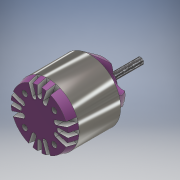
# Autodesk Inventor part: silnik
Saved by Autodesk Inventor 2017 (Build 210142000, 142)
## iProperties
Created: 2016-12-26
Part Number: silnik
Material: Ogólny
Document SubType Name: Modeling
Designer: Kuba01
Density: 1 g/cm^3
Appearance: Domyślna
Author: Kuba01
Autodesk Inventor part; units mm, degrees
ref_plane "YZ Plane" through (0, 0, 0) normal (1, 0, 0) x (0, 1, 0)
ref_plane "XZ Plane" through (0, 0, 0) normal (0, 1, 0) x (-1, 0, 0)
ref_plane "XY Plane" through (0, 0, 0) normal (0, 0, 1) x (1, 0, 0)
sketch "Szkic1" plane through (0, 0, 0) normal (0, 0, 1) x (1, 0, 0)
  line L0 (0, -24.0594) -> (0, 52.0933) projected
  line L1 (0, 38.3467) -> (0, -13.1804)
  line L2 (0, -4.7857) -> (-13, -4.7857)
  line L3 (-13, -4.7857) -> (-14, -0.7857)
  line L4 (-14, -0.7857) -> (-14, 18.2143)
  line L5 (-14, 18.2143) -> (-10, 24.2143)
  line L6 (-10, 24.2143) -> (-4.5, 24.2143)
  line L7 (-4.5, 26.2143) -> (-1.5, 26.2143)
  line L8 (-1.5, 26.2143) -> (-1.5, 41.2143)
  line L9 (-1.5, 41.2143) -> (0, 41.2143)
  line L10 (-4.5, 24.2143) -> (-4.5, 26.2143)
  point P0 (0, 0)
  dimension "d2" = 14
  dimension "d3" = 13
  dimension "d4" = 4
  dimension "d5" = 6
  dimension "d6" = 19
  dimension "d7" = 20
  dimension "d9" = 3
  dimension "d10" = 15
  dimension "d12" = 2
  dimension "d13" = 9
  constraints: 20 end point, 4 point on line, 3 perpendicular, 2 parallel, 1 horizontal, 1 vertical
  measures "d2" distance between parallel lines of L4 L0
  measures "d3" distance of L2.start L2.end
  measures "d4" distance from line of L3.end L2
  measures "d5" distance from line of L6 L4.end
  measures "d6" distance of L3.end L4.end
  measures "d7" diameter of L5.end L1
  measures "d9" diameter of L8 L1
  measures "d10" distance between parallel lines of L9 L7
  measures "d12" distance between parallel lines of L6 L7
  measures "d13" diameter of L10 L1
revolve "Obrót1" add sketch "Szkic1" angle 360 about axis through (0, 38.3467, 0) along (0, -1, 0)
sketch "Szkic2" plane through (0, -4.7857, 0) normal (0, -1, 0) x (1, 0, 0)
  arc A0 (-9, -1) -> (-9, 1) centre (-9, 0) ccw
  line L0 (-9, 1) -> (-12.9615, 1)
  line L1 (-9, -1) -> (-12.9615, -1)
  line L2 (0, 0) -> (-12.3693, 4) construction
  arc A1 (-7.9292, 1.5132) -> (-7.2946, 3.4099) centre (-7.6119, 2.4615) ccw
  line L3 (-12.6285, 3.0855) -> (-7.9292, 1.5132)
  line L4 (-7.2946, 3.4099) -> (-12.0058, 4.9861)
  line L5 (-22.3692, 0) -> (20.0615, 0) projected
  arc A2 (-7.2946, -3.4099) -> (-7.9292, -1.5132) centre (-7.6119, -2.4615) ccw
  line L6 (-12.6285, -3.0855) -> (-7.9292, -1.5132)
  line L7 (-7.2946, -3.4099) -> (-12.0058, -4.9861)
  line L8 (-3.4099, -7.2946) -> (-4.9861, -12.0058)
  arc A3 (-1.5132, -7.9292) -> (-3.4099, -7.2946) centre (-2.4615, -7.6119) ccw
  line L9 (-3.0855, -12.6285) -> (-1.5132, -7.9292)
  line L10 (-1, -9) -> (-1, -12.9615)
  arc A4 (1, -9) -> (-1, -9) centre (0, -9) ccw
  line L11 (1, -9) -> (1, -12.9615)
  line L12 (3.0855, -12.6285) -> (1.5132, -7.9292)
  arc A5 (3.4099, -7.2946) -> (1.5132, -7.9292) centre (2.4615, -7.6119) ccw
  line L13 (3.4099, -7.2946) -> (4.9861, -12.0058)
  line L14 (7.2946, -3.4099) -> (12.0058, -4.9861)
  arc A6 (7.9292, -1.5132) -> (7.2946, -3.4099) centre (7.6119, -2.4615) ccw
  line L15 (12.6285, -3.0855) -> (7.9292, -1.5132)
  line L16 (9, -1) -> (12.9615, -1)
  arc A7 (9, 1) -> (9, -1) centre (9, 0) ccw
  line L17 (9, 1) -> (12.9615, 1)
  line L18 (12.6285, 3.0855) -> (7.9292, 1.5132)
  arc A8 (7.2946, 3.4099) -> (7.9292, 1.5132) centre (7.6119, 2.4615) ccw
  line L19 (7.2946, 3.4099) -> (12.0058, 4.9861)
  line L20 (3.4099, 7.2946) -> (4.9861, 12.0058)
  arc A9 (1.5132, 7.9292) -> (3.4099, 7.2946) centre (2.4615, 7.6119) ccw
  line L21 (3.0855, 12.6285) -> (1.5132, 7.9292)
  line L22 (1, 9) -> (1, 12.9615)
  arc A10 (-1, 9) -> (1, 9) centre (0, 9) ccw
  line L23 (-1, 9) -> (-1, 12.9615)
  line L24 (-3.0855, 12.6285) -> (-1.5132, 7.9292)
  arc A11 (-3.4099, 7.2946) -> (-1.5132, 7.9292) centre (-2.4615, 7.6119) ccw
  line L25 (-3.4099, 7.2946) -> (-4.9861, 12.0058)
  arc A12 (-12.6285, -3.0855) -> (-12.5891, -3.2428) centre (0, 0) ccw
  arc A13 (-4.9861, -12.0058) -> (-3.0855, -12.6285) centre (0, 0) ccw
  arc A14 (-1, -12.9615) -> (1, -12.9615) centre (0, 0) ccw
  arc A15 (3.0855, -12.6285) -> (4.9861, -12.0058) centre (0, 0) ccw
  arc A16 (12.0058, -4.9861) -> (12.6285, -3.0855) centre (0, 0) ccw
  arc A17 (12.9615, -1) -> (12.9615, 1) centre (0, 0) ccw
  arc A18 (12.6285, 3.0855) -> (12.0058, 4.9861) centre (0, 0) ccw
  arc A19 (4.9861, 12.0058) -> (3.0855, 12.6285) centre (0, 0) ccw
  arc A20 (1, 12.9615) -> (-1, 12.9615) centre (0, 0) ccw
  arc A21 (-3.0855, 12.6285) -> (-4.9861, 12.0058) centre (0, 0) ccw
  line L26 (-12.0058, 4.9861) -> (-15.0727, 6.0122)
  line L27 (-15.0727, 6.0122) -> (-15.7072, 4.1156)
  line L28 (-15.7072, 4.1156) -> (-12.6285, 3.0855)
  line L29 (-12.9615, 1) -> (-16.3077, 1)
  line L30 (-16.3077, 1) -> (-16.3077, -1)
  line L31 (-16.3077, -1) -> (-12.9615, -1)
  line L32 (-12.6285, -3.0855) -> (-16.0368, -4.2258)
  line L33 (-16.0368, -4.2258) -> (-15.4022, -6.1225)
  line L34 (-15.4022, -6.1225) -> (-12.0058, -4.9861)
  dimension "d15" = 2
  dimension "d16" = 9
  dimension "d18" = 2
  dimension "d20" = 8
  dimension "d23" = 360
  constraints: 68 end point, 44 point on circle, 22 centre point, 5 perpendicular, 5 symmetric about line, 3 collinear, 2 horizontal, 2 parallel, 2 point on line, 2 tangent, 1 coincident, 1 horizontal alignment, 98 other
  measures "d15" diameter of A0
  measures "d16" distance of A0.centre point (0, 0)
  measures "d18" diameter of A1
  measures "d20" distance of point (0, 0) A1.centre
extrude "Wyciągnięcie proste2" cut sketch "Szkic2" against normal blind 4 contours L1 L31 L30 L5 A0 | L5 L30 L29 L0 A0 | L3 L28 L27 L26 L4 A1 | L7 L34 L33 L32 L6 A2
pattern_circular "Szyk kołowy1" count 4 over 360 about axis through (0, -10, 0) along (0, 1, 0) of "Wyciągnięcie proste2"
sketch "Szkic3" plane through (-12.9615, -4.7857, 1) normal (0, -1, 0) x (1, 0, 0)
  line L0 (9.5516, 6.2946) -> (7.9754, 11.0058) projected
  line L1 (0.9557, 3.9861) -> (5.6669, 2.4099) projected
  line L2 (13.9615, 11.9615) -> (13.9615, 8) projected
  line L3 (11.9615, 8) -> (11.9615, 11.9615) projected
  line L4 (12.9615, -1) -> (12.9615, 11.9615) construction
  circle A0 centre (12.9615, -1) radius 1.5 construction
  line L5 (12.9615, -1) -> (6.244, 5.7175) construction
  dimension "d32" = 9.5
  dimension "d33" = 45
  constraints: 4 end point, 1 vertical
  measures "d32" distance of L5.end L4.start
  measures "d33" angle of L4 L5
hole "Otwór1" at (-6.7175, -4.7857, 6.7175) direction (0, 1, 0) diameter 2.459 depth 4 tip angle 118 thread size "M3x0.5" class "6H" standard "ANSI Metric M Profile"
pattern_circular "Szyk kołowy2" count 4 over 360 about axis through (0, -10, 0) along (0, 1, 0) of "Otwór1"
sketch "Szkic4" plane through (0, 24.2143, 0) normal (0, 1, 0) x (1, 0, 0)
  circle A0 centre (0, 0) radius 4.5 projected
  circle A1 centre (0, 0) radius 14 projected
  arc A2 (13.0646, -7.9311) -> (4.5, -6) centre (9, -6) ccw
  line L0 (-19.6, 0) -> (19.6, 0) projected
  line L1 (0, 19.6) -> (0, -19.6) projected
  line L2 (4.5, 0) -> (4.5, -15.4708) construction
  circle A3 centre (0, 0) radius 10 projected
  line L3 (4.5, -6) -> (4.5, -8.9303) construction
  line L4 (4.5, -8.9303) -> (2.303, -13.8093) construction
  line L5 (2.303, -13.8093) -> (-5.0421, -16.4208) construction
  spline S0 degree 3 poles (4.5, -6) (4.5, -8.9303) (2.303, -13.8093) (-5.0421, -16.4208) knots 1 1 1 1 2 2 2 2
  line L6 (13.0646, -7.9311) -> (9.0312, -16.4208)
  line L7 (9.0312, -16.4208) -> (-5.0421, -16.4208)
  dimension "d44" = 9
  dimension "d45" = 6
  constraints: 6 end point, 3 point on circle, 3 point on line, 2 tangent, 2 vertical, 1 centre point, 1 horizontal, 1 horizontal alignment, 9 other
  measures "d44" diameter of A2
  measures "d45" distance from line of L0 A2.centre
extrude "Wyciągnięcie proste3" cut sketch "Szkic4" against normal blind 6 contours A3 S0 A2 | A2 A1 L1 S0 A3 | L1 A1 S0 | A2 L6 L7 L1 A1 | L1 L7 S0 A1
pattern_circular "Szyk kołowy3" count 4 over 360 about axis through (0, -10, 0) along (0, 1, 0) of "Wyciągnięcie proste3"
